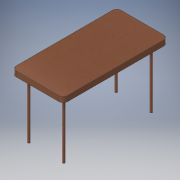
# Autodesk Inventor part: table
Saved by Autodesk Inventor 2017 (Build 210142000, 142)
## iProperties
Created: 2019-04-12
Part Number: table
Material: Wood (Oak)
Document SubType Name: Modeling
Designer: Brian
Density: 0.76 g/cm^3
Appearance: White Oak - Natural Medium Gloss
Author: Brian
Autodesk Inventor part; units mm, degrees
ref_plane "YZ Plane" through (0, 0, 0) normal (1, 0, 0) x (0, 1, 0)
ref_plane "XZ Plane" through (0, 0, 0) normal (0, 1, 0) x (-1, 0, 0)
ref_plane "XY Plane" through (0, 0, 0) normal (0, 0, 1) x (1, 0, 0)
sketch "Sketch1" plane through (0, 0, 0) normal (0, 1, 0) x (-1, 0, 0)
  line L0 (50.8, 0) -> (546.1, 0)
  line L1 (596.9, -50.8) -> (596.9, -1168.4)
  line L2 (546.1, -1219.2) -> (50.8, -1219.2)
  line L3 (0, -1168.4) -> (0, -50.8)
  arc A0 (596.9, -50.8) -> (546.1, 0) centre (546.1, -50.8) ccw
  arc A1 (50.8, 0) -> (0, -50.8) centre (50.8, -50.8) ccw
  arc A2 (0, -1168.4) -> (50.8, -1219.2) centre (50.8, -1168.4) ccw
  arc A3 (546.1, -1219.2) -> (596.9, -1168.4) centre (546.1, -1168.4) ccw
  point P0 (0, 0)
  point P1 (596.9, -1219.2)
  point P2 (596.9, 0)
  point P3 (0, -1219.2)
  dimension "d0" = 596.9
  dimension "d1" = 1219.2
  dimension "d2" = 50.8
  constraints: 8 end point, 8 point on circle, 8 point on line, 8 tangent, 4 centre point, 3 equal radius, 2 parallel, 1 horizontal, 1 perpendicular
  measures "d0" distance of point (596.9, -1219.2) point (0, -1219.2)
  measures "d1" distance of point (596.9, 0) point (596.9, -1219.2)
  measures "d2" radius of A0
extrude "Extrusion1" add sketch "Sketch1" along normal blind 63.5
sketch "Sketch2" plane through (0, 0, 0) normal (0, -1, 0) x (1, 0, 0)
  circle A0 centre (-95.25, -101.6) radius 12.7
  line L0 (-222.0778, -191.3187) -> (-285.2767, -191.3187) construction
  circle A1 centre (-501.65, -101.6) radius 12.7
  line L1 (0, -50.8) -> (0, -1168.4) projected
  line L2 (-596.9, -1168.4) -> (-596.9, -50.8) projected
  line L3 (-50.8, -1219.2) -> (-546.1, -1219.2) projected
  line L4 (-546.1, 0) -> (-50.8, 0) projected
  circle A2 centre (-95.25, -1117.6) radius 12.7
  circle A3 centre (-501.65, -1117.6) radius 12.7
  point P0 (0, 0)
  dimension "d5" = 12.7
  dimension "d8" = 406.4
  dimension "d13" = 95.25
  dimension "d15" = 95.25
  dimension "d16" = 596.9
  dimension "d17" = 1219.2
  dimension "d18" = 101.6
  dimension "d21" = 1016
  dimension "d26" = 101.6
  constraints: 4 centre point, 2 end point, 1 horizontal, 1 vertical, 6 other
  measures "d5" radius of A0
  measures "d8" distance of A0.centre A1.centre
  measures "d13" distance from line of L1 A0.centre
  measures "d15" distance from line of L2 A1.centre
  measures "d16" distance between parallel lines of L2 L1
  measures "d17" distance between parallel lines of L3 L4
  measures "d18" distance from line of A0.centre L4
  measures "d21" distance of A0.centre A2.centre
  measures "d26" distance from line of A2.centre L3
extrude "Extrusion2" add sketch "Sketch2" along normal blind 685.8 separate body
equation "\"d13\" = d15"
equation "\"d15\" = 0.5 * d16 - 0.5 * d8"
equation "\"d18\" = 0.0833333 * d17"
equation "\"d26\" = d18"
body "Solid1"
body "Solid2"
